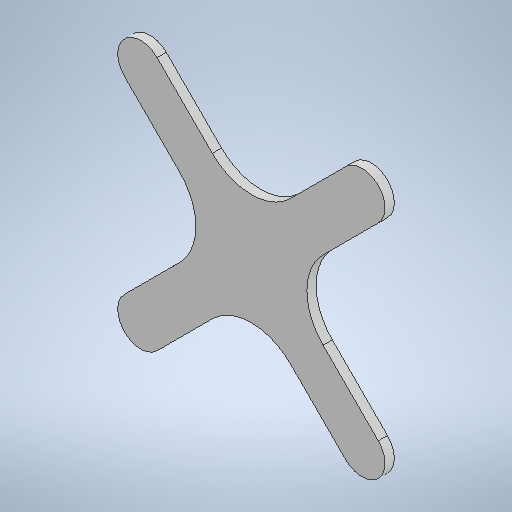
# Autodesk Inventor part: Base
Saved by Autodesk Inventor 2025.1 (Build 291241020, 241B)
## iProperties
Created: 2024-09-22
Part Number: Base
Material: 일반
Document SubType Name: Modeling
Designer: daare
Density: 1 g/cm^3
Appearance: 기본값
Author: daare
Autodesk Inventor part; units mm, degrees
ref_plane "YZ Plane" through (0, 0, 0) normal (1, 0, 0) x (0, 1, 0)
ref_plane "XZ Plane" through (0, 0, 0) normal (0, 1, 0) x (-1, 0, 0)
ref_plane "XY Plane" through (0, 0, 0) normal (0, 0, 1) x (1, 0, 0)
sketch "스케치1" plane through (0, 0, 0) normal (0, 0, 1) x (1, 0, 0)
  arc A0 (-51.1612, 68.8388) -> (-68.8388, 51.1612) centre (-60, 60) ccw
  line L0 (-68.8388, 51.1612) -> (-38.8909, 21.2132)
  line L1 (-51.1612, 68.8388) -> (-21.2132, 38.8909)
  line L2 (-60, 60) -> (0, 0)
  arc A1 (-30.1041, 0) -> (-38.8909, 21.2132) centre (-60.1041, 0) ccw
  line L3 (-93.2132, 0) -> (15.5355, 0) projected
  arc A2 (-21.2132, 38.8909) -> (0, 30.1041) centre (0, 60.1041) ccw
  line L4 (0, -15.5355) -> (0, 93.2132) projected
  dimension "d0" = 60
  dimension "d1" = 60
  dimension "d2" = 25
  dimension "d3" = 30
  constraints: 6 end point, 6 point on circle, 3 centre point, 3 symmetric about line, 3 tangent, 2 parallel, 1 horizontal alignment, 1 point on line, 1 other
  measures "d0" horizontal distance of L2.end L2.start
  measures "d1" horizontal distance of L2.end L2.start
  measures "d2" diameter of A0
  measures "d3" radius of A1
extrude "돌출1" add sketch "스케치1" along normal blind 5
pattern_circular "원형 패턴1" count 4 over 360 about axis through (0, 0, -10) along (0, 0, 1) of "돌출1"
